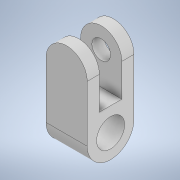
# Autodesk Inventor part: 16
Saved by Autodesk Inventor 2022 (Build 260153000, 153)
## iProperties
Created: 2022-03-14
Part Number: 16
Material: Všeobecné
Document SubType Name: Modeling
Designer: Šimon
Density: 1 g/cm^3
Appearance: Výchozí
Author: Šimon
Autodesk Inventor part; units mm, degrees
ref_plane "YZ Plane" through (0, 0, 0) normal (1, 0, 0) x (0, 1, 0)
ref_plane "XZ Plane" through (0, 0, 0) normal (0, 1, 0) x (-1, 0, 0)
ref_plane "XY Plane" through (0, 0, 0) normal (0, 0, 1) x (1, 0, 0)
sketch "Náčrt3" plane through (0, 0, 0) normal (0, 0, 1) x (1, 0, 0)
  arc A0 (22, 0) -> (-22, 0) centre (0, 0) ccw
  line L0 (-22, 0) -> (-22, -60)
  line L1 (22, 0) -> (22, -60)
  line L2 (-22, -60) -> (22, -60)
  dimension "d15" = 44
  dimension "d16" = 60
  dimension "d17" = 60
  constraints: 6 end point, 2 point on circle, 2 vertical, 1 centre point, 1 horizontal, 1 tangent
  measures "d15" diameter of A0
  measures "d16" distance of L0.start L0.end
  measures "d17" distance of L1.start L1.end
extrude "Vysunutí3" add sketch "Náčrt3" along normal blind 50
sketch "Náčrt4" plane through (22, -60, 0) normal (1, 0, 0) x (0, 0, -1)
  line L0 (0, 0) -> (-50, 0) projected
  circle A0 centre (-25, 0) radius 25
  circle A1 centre (-25, 0) radius 15
  point P0 (0, 60)
  dimension "d20" = 50
  dimension "d21" = 30
  constraints: 2 centre point, 1 coincident, 1 midpoint
  measures "d20" diameter of A0
  measures "d21" diameter of A1
extrude "Vysunutí4" add sketch "Náčrt4" against normal blind 44 contours A0 L0 A1 | L0 A1 A0
sketch "Náčrt5" plane through (-22, 0, 0) normal (-1, 0, 0) x (0, 0, 1)
  line L0 (13, -35) -> (37, -35)
  line L1 (37, -35) -> (37, 53.1148)
  line L2 (37, 53.1148) -> (13, 53.1148)
  line L3 (13, 53.1148) -> (13, -35)
  line L4 (50, 0) -> (50, -60) projected
  arc A0 (0, -60) -> (50, -60) centre (25, -60) ccw projected
  circle A1 centre (25, -60) radius 15
  point P0 (0, 0)
  dimension "d24" = 24
  dimension "d25" = 13
  dimension "d27" = 50
  constraints: 8 end point, 2 parallel, 1 centre point, 1 coincident, 1 horizontal, 1 perpendicular
  measures "d24" distance between parallel lines of L1 L3
  measures "d25" distance between parallel lines of L4 L1
extrude "Vysunutí5" cut sketch "Náčrt5" against normal through all
sketch "Náčrt6" plane through (0, 0, 0) normal (0, 0, -1) x (-1, 0, 0)
  circle A0 centre (0, 0) radius 10
  dimension "d30" = 20
  constraints: 1 centre point, 1 coincident
  measures "d30" diameter of A0
extrude "Vysunutí6" cut sketch "Náčrt6" against normal blind 20
equation "\"d31\" = d30"
